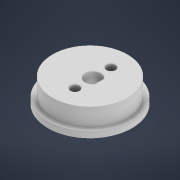
# Autodesk Inventor part: InputShaft2
Saved by Autodesk Inventor 2022 (Build 260153000, 153)
## iProperties
Created: 2022-10-09
Part Number: InputShaft2
Material: Ogólny
Document SubType Name: Modeling
Designer: MicnedSQ
Density: 1 g/cm^3
Appearance: Domyślna
Author: MicnedSQ
## iProperties of the stored document InputShaft2_3DPrint.ipt
Created: 2022-10-19
Part Number: InputShaft2_3DPrint
Material: Generic
Document SubType Name: Modeling
Designer: MicnedSQ
Density: 1 g/cm^3
Appearance: Default
Author: MicnedSQ
Autodesk Inventor part; units mm, degrees
ref_plane "YZ Plane" through (0, 0, 0) normal (1, 0, 0) x (0, 1, 0)
ref_plane "XZ Plane" through (0, 0, 0) normal (0, 1, 0) x (-1, 0, 0)
ref_plane "XY Plane" through (0, 0, 0) normal (0, 0, 1) x (1, 0, 0)
sketch "Szkic1" plane through (0, 0, 0) normal (0, 1, 0) x (-1, 0, 0)
  circle A0 centre (0, 0) radius 14
  dimension "d0" = 28
  constraints: 1 centre point, 1 coincident
  measures "d0" diameter of A0
extrude "Wyciągnięcie proste1" add sketch "Szkic1" along normal blind 2
sketch "Szkic2" plane through (0, 2, 0) normal (0, 1, 0) x (1, 0, 0)
  circle A0 centre (0, 0) radius 12.5
  dimension "d3" = 25
  constraints: 1 centre point, 1 coincident
  measures "d3" diameter of A0
extrude "Wyciągnięcie proste2" add sketch "Szkic2" along normal blind 6
sketch "Szkic3" plane through (0, 8, 0) normal (0, 1, 0) x (1, 0, 0)
  circle A0 centre (1, -6) radius 1.5
  point P0 (0, 0)
  dimension "d6" = 3
  dimension "d10" = 6
  dimension "d11" = 1
  constraints: 1 centre point
  measures "d6" diameter of A0
  measures "d10" vertical distance of A0.centre point (0, 0)
  measures "d11" horizontal distance of A0.centre point (0, 0)
extrude "Wyciągnięcie proste3" cut sketch "Szkic3" against normal up to surface (8 mm away)
mirror "Odbij1" about plane through (0, 0, 0) normal (0, 0, 1) of "Wyciągnięcie proste3"
sketch "Sketch5" plane through (0, 8, 0) normal (0, 1, 0) x (1, 0, 0)
  arc A0 (3.12, 1.59) -> (3.12, -1.59) centre (1, 0) ccw
  line L0 (3.12, -1.59) -> (3.12, 1.59)
  point P0 (0, 0)
  dimension "d12" = 5.3
  dimension "d13" = 3.18
  dimension "d14" = 1
  dimension "d15" = 0
  constraints: 2 end point, 2 point on circle, 1 centre point, 1 vertical
  measures "d12" diameter of A0
  measures "d13" distance of L0.start L0.end
  measures "d14" distance of point (0, 0) A0.centre
  measures "d15" vertical distance of point (0, 0) A0.centre
extrude "Extrusion4" cut sketch "Sketch5" against normal up to surface (8 mm away)
